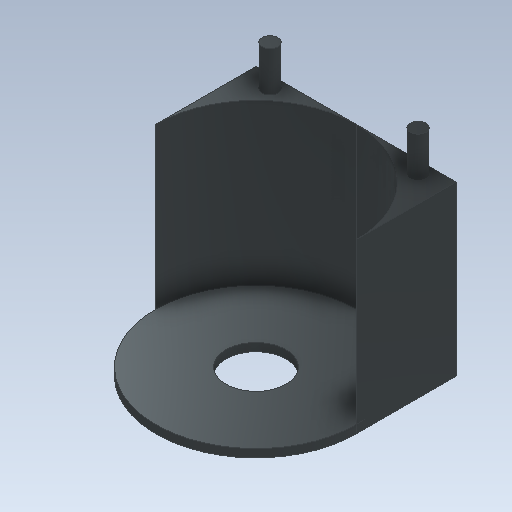
# Autodesk Inventor part: trail 3.1
Saved by Autodesk Inventor 2020.2 (Build 242310000, 310)
## iProperties
Created: 2020-02-17
Part Number: trail 3.1
Material: Iron, Gray
Document SubType Name: Modeling
Designer: lenovo
Density: 7.15 g/cm^3
Appearance: Iron Gray
Author: lenovo
Autodesk Inventor part; units mm, degrees
ref_plane "YZ Plane" through (0, 0, 0) normal (1, 0, 0) x (0, 1, 0)
ref_plane "XZ Plane" through (0, 0, 0) normal (0, 1, 0) x (-1, 0, 0)
ref_plane "XY Plane" through (0, 0, 0) normal (0, 0, 1) x (1, 0, 0)
sketch "Sketch1" plane through (0, 0, 0) normal (0, 1, 0) x (-1, 0, 0)
  circle A0 centre (0, 0) radius 7.5
  circle A1 centre (0, 0) radius 25
  dimension "d0" = 15
  dimension "d1" = 50
  constraints: 2 centre point, 2 coincident
  measures "d0" diameter of A0
  measures "d1" diameter of A1
extrude "Extrusion1" add sketch "Sketch1" along normal blind 2
sketch "Sketch2" plane through (0, 2, 0) normal (0, 1, 0) x (1, 0, 0)
  circle A0 centre (0, 0) radius 25 projected
  line L0 (25, 0) -> (-25, 0)
  line L1 (-25, 0) -> (-25, 25)
  line L2 (-25, 25) -> (25, 25)
  line L3 (25, 25) -> (25, 0)
  point P0 (0, 25)
  constraints: 8 end point, 2 parallel, 1 horizontal, 1 perpendicular, 2 other
extrude "Extrusion2" add sketch "Sketch2" along normal blind 10 and the other way blind 2 contours L1 L2 A0 | A0 L2 L3
sketch "Sketch3" plane through (0, 12, 0) normal (0, 1, 0) x (1, 0, 0)
  circle A0 centre (21.5, 18.5) radius 2
  circle A1 centre (-21.5, 18.5) radius 2
  point P0 (0, 0)
  dimension "d8" = 4
  dimension "d9" = 4
  constraints: 2 centre point
  measures "d8" diameter of A0
  measures "d9" diameter of A1
extrude "Extrusion3" add sketch "Sketch3" along normal blind 40
sketch "Sketch4" plane through (0, 0, 0) normal (0, -1, 0) x (1, 0, 0)
  line L0 (25, -25) -> (0, -25) projected
  arc A0 (25, 0) -> (-25, 0) centre (0, 0) ccw projected
  line L1 (25, -25) -> (-25, -25)
  line L2 (-25, -25) -> (-25, 0)
  line L3 (-25, 0) -> (25, 0)
  line L4 (25, 0) -> (25, -25)
  arc A1 (0, -25) -> (25, 0) centre (0, 0) ccw projected
  arc A2 (-25, 0) -> (25, 0) centre (0, 0) ccw
  constraints: 8 end point, 3 point on circle, 2 parallel, 1 centre point, 1 concentric, 1 horizontal, 1 perpendicular
extrude "Extrusion4" add sketch "Sketch4" against normal blind 42 contours L0 A1 L4 | L1 L2 A2
sketch "Sketch5" plane through (21.5, 52, -18.5) normal (0, 1, 0) x (1, 0, 0)
  circle A0 centre (0, 0) radius 2 projected
  circle A1 centre (0, 0) radius 2
  circle A2 centre (-43, 0) radius 2 projected
  circle A3 centre (-43, 0) radius 2
  point P0 (-21.5, -18.5)
  constraints: 2 centre point, 2 coincident
extrude "Extrusion5" cut sketch "Sketch5" against normal blind 10
sketch "Sketch6" plane through (0, 42, 0) normal (0, 1, 0) x (1, 0, 0)
  circle A0 centre (18.5, 22) radius 2
  circle A1 centre (-18.5, 22) radius 2
  point P0 (0, 0)
  dimension "d16" = 4
  dimension "d17" = 4
  constraints: 2 centre point
  measures "d16" diameter of A0
  measures "d17" diameter of A1
extrude "Extrusion6" add sketch "Sketch6" along normal blind 10
body "Solid1"
